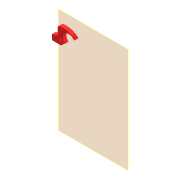
# Autodesk Inventor part: 30_xystage_gp-010b_adapter_multiwellplate_flexureclamp
Saved by Autodesk Inventor 2022 (Build 260153000, 153)
## iProperties
Created: 2023-06-04
Part Number: 30_xystage_gp-010b_adapter_multiwellplate_flexureclamp
Material: Generisch
Document SubType Name: Modeling
Designer: diederichbenedict
Density: 1 g/cm^3
Appearance: Hellrot
Author: diederichbenedict
Autodesk Inventor part; units mm, degrees
ref_plane "YZ Plane" through (0, 0, 0) normal (1, 0, 0) x (0, 1, 0)
ref_plane "XZ Plane" through (0, 0, 0) normal (0, 1, 0) x (-1, 0, 0)
ref_plane "XY Plane" through (0, 0, 0) normal (0, 0, 1) x (1, 0, 0)
ref_plane "Arbeitsebene1" through (0, 0, 0) normal (0, 0, 1) x (1, 0, 0)
sketch "Skizze1" plane through (0, 0, 0) normal (0, 0, 1) x (1, 0, 0)
  line L0 (-43.5249, 65.0249) -> (-30, 65.0249) projected
  line L1 (-43.5249, -65.0249) -> (-43.5249, 65.0249) projected
  circle A0 centre (-50, 52.5) radius 1.4 projected
  line L2 (-46, 72.5) -> (-50, 72.5)
  line L3 (-55, 67.5) -> (-55, 59.5)
  line L4 (-55, 44.5) -> (-51, 44.5)
  line L5 (-46, 49.5) -> (-46, 58.0276)
  line L6 (-55, 44.5) -> (-70, 44.5)
  line L7 (-70, 44.5) -> (-70, 54.5)
  line L8 (-70, 54.5) -> (-60, 54.5)
  line L9 (-55, 54.5) -> (-55, 44.5)
  circle A1 centre (-50, 52.5) radius 1.6
  arc A2 (-25.9255, 64.7266) -> (-46, 72.5) centre (-46, 42.6923) ccw
  arc A3 (-26.9357, 63.6178) -> (-30.5378, 66.404) centre (-46, 42.6923) ccw
  arc A4 (-30.5378, 66.404) -> (-46, 58.0276) centre (-36, 58.0276) ccw
  arc A5 (-26.9357, 63.6178) -> (-25.9255, 64.7266) centre (-26.4306, 64.1722) ccw
  arc A6 (-46, 58.0276) -> (-42.9999, 50.8861) centre (-36, 58.0276) ccw
  arc A7 (-46, 52.3487) -> (-44.0499, 49.8149) centre (-36, 58.0276) ccw
  arc A8 (-44.0499, 49.8149) -> (-42.9999, 50.8861) centre (-43.5249, 50.3505) ccw
  arc A9 (-51, 44.5) -> (-46, 49.5) centre (-51, 49.5) ccw
  arc A10 (-60, 54.5) -> (-55, 59.5) centre (-60, 59.5) ccw
  arc A11 (-50, 72.5) -> (-55, 67.5) centre (-50, 67.5) ccw
  point P0 (0, 0)
  point P1 (-55, 72.5)
  point P2 (-46, 44.5)
  point P3 (-27.3644, 64.0006)
  point P4 (-46, 71)
  dimension "d0" = 4
  dimension "d1" = 5
  dimension "d2" = 8
  dimension "d3" = 10
  dimension "d4" = 15
  dimension "d5" = 20
  dimension "d6" = 3.2
  dimension "d10" = 1.5
  dimension "d12" = 10
  dimension "d13" = 0.75
  dimension "d14" = 1.5
  dimension "d15" = 5
  constraints: 23 point on circle, 16 end point, 13 tangent, 11 centre point, 10 point on line, 4 parallel, 3 equal radius, 2 coincident, 2 horizontal, 2 perpendicular, 1 concentric
  measures "d0" distance from line of L5 A0.centre
  measures "d1" distance from line of L3 A0.centre
  measures "d2" distance from line of A0.centre L4
  measures "d3" distance between parallel lines of L8 L6
  measures "d4" distance between parallel lines of L3 L7
  measures "d5" distance from line of A0.centre L2
  measures "d6" diameter of A1
  measures "d10" radial gap between concentric circles of A2 A3
  measures "d12" radius of A4
  measures "d13" radius of A5
  measures "d14" radial gap between concentric circles of A6 A7
  measures "d15" radius of A9
extrude "Extrusion1" add sketch "Skizze1" along normal blind 6 contours L1 A4 L5 A9 L4 L6 L7 L8 A10 L3 A11 L2 A2 A5 A3 L0 | L0 A4 L1 | A6 A8 L1 | L1 A8 A7 L5 A6
fillet "Rundung1" radius 2 3 edges at (-70, 54.5, 3) (-70, 44.5, 3) (-46, 72.5, 3)
sketch "Skizze2" plane through (0, 0, 0) normal (0, 0, -1) x (-1, 0, 0)
  line L0 (70, 52.5) -> (70, 46.5) projected
  arc A0 (68, 44.5) -> (70, 46.5) centre (68, 46.5) ccw projected
  line L1 (68, 44.5) -> (51, 44.5) projected
  arc A1 (46, 49.5) -> (51, 44.5) centre (51, 49.5) ccw projected
  line L2 (46, 49.5) -> (46, 52.3487) projected
  arc A2 (44.0499, 49.8149) -> (46, 52.3487) centre (36, 58.0276) ccw projected
  arc A3 (42.9999, 50.8861) -> (44.0499, 49.8149) centre (43.5249, 50.3505) ccw projected
  arc A4 (42.9999, 50.8861) -> (30.5378, 66.404) centre (36, 58.0276) ccw projected
  arc A5 (30.5378, 66.404) -> (26.9357, 63.6178) centre (46, 42.6923) ccw projected
  arc A6 (25.9255, 64.7266) -> (26.9357, 63.6178) centre (26.4306, 64.1722) ccw projected
  arc A7 (46, 72.5) -> (25.9255, 64.7266) centre (46, 42.6923) ccw projected
  line L3 (46, 72.5) -> (50, 72.5) projected
  arc A8 (55, 67.5) -> (50, 72.5) centre (50, 67.5) ccw projected
  line L4 (55, 67.5) -> (55, 59.5) projected
  arc A9 (55, 59.5) -> (60, 54.5) centre (60, 59.5) ccw projected
  line L5 (60, 54.5) -> (68, 54.5) projected
  arc A10 (70, 52.5) -> (68, 54.5) centre (68, 52.5) ccw projected
  line L6 (70, 52.5) -> (70, 46.5) projected
  circle A11 centre (50, 52.5) radius 1.6 projected
  line L7 (64, 54.5) -> (64, 44.5)
  point P0 (0, 0)
  dimension "d16" = 6
  constraints: 2 end point, 1 midpoint, 1 parallel, 1 perpendicular, 1 point on line
  measures "d16" distance between parallel lines of L0 L7
extrude "Extrusion2" add sketch "Skizze2" along normal blind 5.5 contours L0 A0 L1 L7 L5 A10
sketch "Skizze3" plane through (-70, 46.5, 6) normal (-1, 0, 0) x (0, 0, 1)
  line L0 (0, 0) -> (-11.5, 0) projected
  line L1 (0, 6) -> (0, 0) projected
  line L2 (0, 6) -> (-11.5, 6) projected
  line L3 (-11.5, 0) -> (-11.5, 6) projected
  circle A0 centre (-8.4091, 3) radius 1.4
  point P0 (-6, -46.5)
  dimension "d19" = 2.8
  constraints: 1 centre point
  measures "d19" diameter of A0
extrude "Extrusion3" cut sketch "Skizze3" against normal through all contours A0
